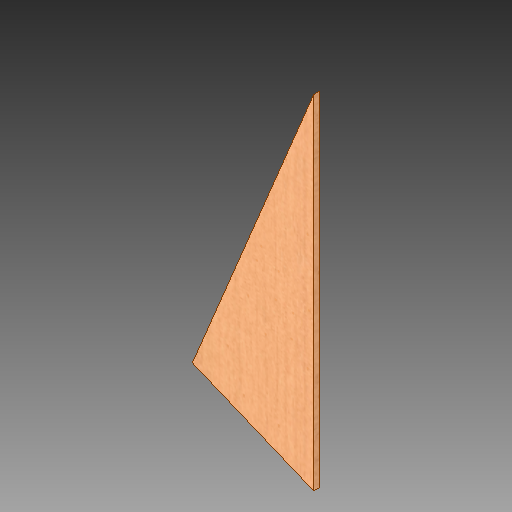
# Autodesk Inventor part: ref1
Saved by Autodesk Inventor 2019 (Build 230136000, 136)
## iProperties
Created: 2019-01-07
Part Number: ref1
Material: Wood (Cherry)
Document SubType Name: Modeling
Designer: gaincarlo
Density: 0.63 g/cm^3
Appearance: Cherry - Natural Low Gloss
Author: gaincarlo
Autodesk Inventor part; units mm, degrees
ref_plane "YZ Plane" through (0, 0, 0) normal (1, 0, 0) x (0, 1, 0)
ref_plane "XZ Plane" through (0, 0, 0) normal (0, 1, 0) x (-1, 0, 0)
ref_plane "Work Plane1" through (0, 0, 0) normal (0, 0, 1) x (1, 0, 0)
sketch "Sketch1" plane through (0, 0, 0) normal (0, 0, 1) x (1, 0, 0)
  line L0 (300, -300) -> (300, 300) construction
  line L1 (303.8268, 63.0866) -> (-250.5009, 292.6966) construction
  line L2 (300, 300) -> (300, 64.6717)
  line L3 (300, 300) -> (216.7989, 99.1347)
  line L4 (300, 64.6717) -> (216.7989, 99.1347)
  point P0 (0, 0)
  constraints: 6 end point, 3 point on line, 1 collinear, 1 perpendicular
extrude "Extrusion1" add sketch "Sketch1" along normal blind 4
body "Solid1"
